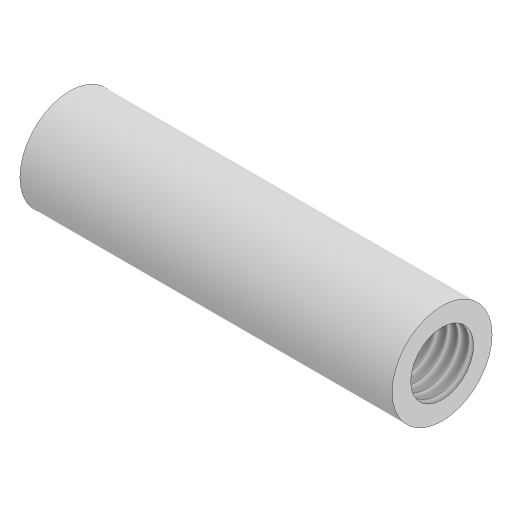
# Autodesk Inventor part: m4 standoff 23.65
Saved by Autodesk Inventor 2023 (Build 270158000, 158)
## iProperties
Created: 2022-11-15
Part Number: m4 standoff 23.65
Material: Generic
Document SubType Name: Modeling
Designer: deli
Density: 1 g/cm^3
Appearance: Default
Author: deli
Autodesk Inventor part; units mm, degrees
ref_plane "YZ Plane" through (0, 0, 0) normal (1, 0, 0) x (0, 1, 0)
ref_plane "XZ Plane" through (0, 0, 0) normal (0, 1, 0) x (-1, 0, 0)
ref_plane "XY Plane" through (0, 0, 0) normal (0, 0, 1) x (1, 0, 0)
sketch "Sketch1" plane through (0, 0, 0) normal (1, 0, 0) x (0, 1, 0)
  circle A0 centre (112.1155, 70.7876) radius 3.175
  circle A1 centre (112.1155, 70.7876) radius 2
  point P0 (0, 0)
  dimension "d0" = 6.35
  dimension "d1" = 4
  constraints: 2 centre point, 1 coincident
  measures "d0" diameter of A0
  measures "d1" diameter of A1
extrude "Extrusion1" add sketch "Sketch1" along normal blind 23.65
thread "Thread1" size "M4x0.7" class "6H" standard "ANSI Metric M Profile" full length
body "Solid1"
